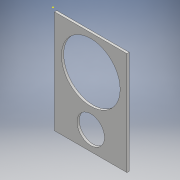
# Autodesk Inventor part: frontal
Saved by Autodesk Inventor 2018 (Build 220112000, 112)
## iProperties
Created: 2019-02-27
Part Number: frontal
Material: Genérico
Document SubType Name: Modeling
Designer: USUARIO WINDOWS
Density: 1 g/cm^3
Appearance: Valor por defecto
Author: USUARIO WINDOWS
Autodesk Inventor part; units mm, degrees
ref_plane "YZ Plane" through (0, 0, 0) normal (1, 0, 0) x (0, 1, 0)
ref_plane "XZ Plane" through (0, 0, 0) normal (0, 1, 0) x (-1, 0, 0)
ref_plane "XY Plane" through (0, 0, 0) normal (0, 0, 1) x (1, 0, 0)
sketch "Boceto1" plane through (0, 0, 0) normal (0, 1, 0) x (-1, 0, 0)
  line L0 (0, 0) -> (-105, 0)
  line L1 (-105, 0) -> (-105, -140)
  line L2 (-105, -140) -> (0, -140)
  line L3 (0, -140) -> (0, 0)
  dimension "d0" = 105
  dimension "d1" = 140
  constraints: 8 end point, 2 parallel, 1 horizontal, 1 perpendicular
  measures "d0" distance of L2.end L1.end
  measures "d1" distance between parallel lines of L2 L0
extrude "Extrusión1" add sketch "Boceto1" along normal blind 3
sketch "Boceto2" plane through (0, 3, 0) normal (0, 1, 0) x (1, 0, 0)
  line L0 (0, 0) -> (105, 0) projected
  line L1 (105, 0) -> (105, 140) projected
  line L2 (105, 140) -> (0, 140) projected
  line L3 (0, 140) -> (0, 0) projected
  circle A0 centre (52.5, 46) radius 38.5
  circle A1 centre (52.5, 111) radius 18
  dimension "d4" = 77
  dimension "d5" = 46
  dimension "d6" = 52.5
  dimension "d7" = 36
  dimension "d8" = 52.5
  dimension "d13" = 65
  constraints: 2 centre point
  measures "d4" diameter of A0
  measures "d5" distance from line of L0 A0.centre
  measures "d6" distance from line of L3 A0.centre
  measures "d7" diameter of A1
  measures "d8" distance from line of L3 A1.centre
  measures "d13" distance of A0.centre A1.centre
extrude "Extrusión2" cut sketch "Boceto2" against normal blind 3 contours A0 | A1
sketch "Boceto3" plane through (0, 0, 0) normal (0, -1, 0) x (1, 0, 0)
  circle A0 centre (52.5, -111) radius 18 projected
  circle A1 centre (52.5, -46) radius 38.5 projected
  line L0 (0, 0) -> (105, 0) projected
  line L1 (0, -140) -> (0, 0) projected
  line L2 (105, -140) -> (0, -140) projected
  line L3 (105, 0) -> (105, -140) projected
  line L4 (105, -140) -> (0, -140) projected
  line L5 (0, -140) -> (0, 0) projected
  line L6 (105, -140) -> (0, -140)
  line L7 (0, -140) -> (0, -136)
  line L8 (0, -136) -> (105, -136)
  line L9 (105, -136) -> (105, -140)
  dimension "d14" = 4
  constraints: 8 end point, 2 parallel, 1 horizontal, 1 perpendicular, 1 point on line
  measures "d14" distance of L6.end L7.end
extrude "Extrusión3" cut sketch "Boceto3" against normal blind 3 contours L8 L3 L2 L1
sketch "Boceto4" plane through (0, 0, 0) normal (0, -1, 0) x (1, 0, 0)
  line L0 (0, -136) -> (105, -136) projected
  line L1 (105, 0) -> (105, -136) projected
  line L2 (0, 0) -> (105, 0) projected
  line L3 (0, -136) -> (0, 0) projected
  circle A0 centre (52.5, -111) radius 18 projected
  circle A1 centre (52.5, -46) radius 38.5 projected
  line L4 (105, -136) -> (0, -136) projected
  line L5 (2.5, 0) -> (102.5, 0)
  line L6 (102.5, 0) -> (102.5, -136)
  line L7 (102.5, -136) -> (2.5, -136)
  line L8 (2.5, -136) -> (2.5, 0)
  line L9 (2.5, 0) -> (102.5, -136) construction
  line L10 (102.5, 0) -> (2.5, -136) construction
  point P0 (52.5, -68)
  dimension "d17" = 100
  constraints: 12 end point, 2 midpoint, 2 parallel, 1 horizontal, 1 perpendicular, 1 point on line
  measures "d17" distance of L6.end L7.end
extrude "Extrusión4" cut sketch "Boceto4" against normal blind 3 contours L3 L2 L8 L0 | L6 L2 L1 L0
sketch "Boceto5" plane through (0, 3, 0) normal (0, 1, 0) x (1, 0, 0)
  point P0 (0, 0)
sketch "Boceto6" plane through (2.5, 0, 0) normal (0, 0, 1) x (1, 0, 0)
  line L0 (0, 3) -> (0, 0) projected
  line L1 (0, 0) -> (100, 0) projected
  line L2 (100, 0) -> (100, 3) projected
  line L3 (0, 3) -> (100, 3) projected
  point P0 (-2.5, 0)
extrude "Extrusión5" cut sketch "Boceto6" against normal blind 1
sketch "Boceto7" plane through (0, 3, 0) normal (0, 1, 0) x (1, 0, 0)
  line L0 (2.5, 1) -> (102.5, 1) projected
  line L1 (102.5, 1) -> (102.5, 136) projected
  line L2 (102.5, 136) -> (2.5, 136) projected
  line L3 (2.5, 136) -> (2.5, 1) projected
  circle A0 centre (52.5, 46) radius 38.5 projected
  circle A1 centre (52.5, 111) radius 18 projected
  line L4 (102.5, 136) -> (2.5, 136) projected
  line L5 (100, 1) -> (5, 1)
  line L6 (5, 1) -> (5, 136)
  line L7 (5, 136) -> (100, 136)
  line L8 (100, 136) -> (100, 1)
  line L9 (100, 1) -> (5, 136) construction
  line L10 (5, 1) -> (100, 136) construction
  point P0 (0, 0)
  point P1 (52.5, 68.5)
  dimension "d22" = 95
  constraints: 12 end point, 2 midpoint, 2 parallel, 1 horizontal, 1 perpendicular, 1 point on line
  measures "d22" distance of L6.end L7.end
extrude "Extrusión6" cut sketch "Boceto7" against normal blind 3 contours L3 L2 L6 L0 | L8 L2 L1 L0
equation "\"d8\" = d6"
